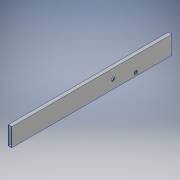
# Autodesk Inventor part: Side Extrusion
Saved by Autodesk Inventor 2019.4 (Build 234330000, 330)
## iProperties
Created: 2019-10-20
Part Number: Side Extrusion
Material: Aluminum 6061
Document SubType Name: Modeling
Designer: Mark
Density: 2.7 g/cm^3
Appearance: Aluminum - Flat
HoleDistanceX: 199.089 mm
Author: Mark
Autodesk Inventor part; units mm, degrees
ref_plane "YZ Plane" through (0, 0, 0) normal (1, 0, 0) x (0, 1, 0)
ref_plane "XZ Plane" through (0, 0, 0) normal (0, 1, 0) x (-1, 0, 0)
ref_plane "XY Plane" through (0, 0, 0) normal (0, 0, 1) x (1, 0, 0)
sketch "Sketch1" plane through (0, 0, 0) normal (0, 0, 1) x (1, 0, 0)
  line L0 (-10, -50) -> (10, -50)
  line L1 (10, -50) -> (10, 50)
  line L2 (10, 50) -> (-10, 50)
  line L3 (-10, 50) -> (-10, -50)
  line L4 (-10, -50) -> (10, 50) construction
  line L5 (10, -50) -> (-10, 50) construction
  line L6 (-8, -48) -> (8, -48)
  line L7 (8, -48) -> (8, 48)
  line L8 (8, 48) -> (-8, 48)
  line L9 (-8, 48) -> (-8, -48)
  line L10 (-8, -48) -> (8, 48) construction
  line L11 (8, -48) -> (-8, 48) construction
  point P0 (0, 0)
  dimension "d0" = 20
  dimension "d1" = 100
  dimension "d2" = 16
  dimension "d3" = 96
  constraints: 24 end point, 4 midpoint, 4 parallel, 2 horizontal, 2 perpendicular
  measures "d0" distance of L2.end L1.end
  measures "d1" distance of L1.end L0.end
  measures "d2" distance of L8.end L7.end
  measures "d3" distance of L7.end L6.end
extrude "Extrusion1" add sketch "Sketch1" along normal blind 880
sketch "Sketch2" plane through (-10, -50, 0) normal (-1, 0, 0) x (0, 0, 1)
  circle A0 centre (199.089, 18.548) radius 9.8
  line L0 (0, 100) -> (880, 100) projected
  line L1 (0, 100) -> (0, 0) projected
  line L2 (0, 0) -> (880, 0) projected
  point P0 (0, 50)
  dimension "d6" = 19.6
  dimension "HoleDistanceX" = 199.089
  dimension "d11" = 18.548
  constraints: 1 centre point
  measures "d6" diameter of A0
  measures "HoleDistanceX" distance from line of L1 A0.centre
  measures "d11" distance from line of L2 A0.centre
extrude "Extrusion2" cut sketch "Sketch2" against normal blind 880
sketch "Sketch4" plane through (-10, -50, 0) normal (-1, 0, 0) x (0, 0, 1)
  circle A0 centre (113.659, 8.082) radius 4.5 construction
  circle A1 centre (199.089, 18.548) radius 8.3 construction
  line L0 (199.089, 18.548) -> (113.659, 8.082) construction
  line L1 (199.089, 18.548) -> (113.0203, 18.5713) construction
  circle A2 centre (113.0203, 18.5713) radius 4.5 construction
  arc A3 (113.0203, 18.5713) -> (113.659, 8.082) centre (199.089, 18.548) ccw construction
  arc A4 (113.0203, 18.5713) -> (113.659, 8.082) centre (199.089, 18.548) ccw construction
  arc A5 (108.5203, 18.5725) -> (109.1924, 7.5348) centre (199.089, 18.548) ccw
  arc A6 (117.5203, 18.5701) -> (118.1256, 8.6292) centre (199.089, 18.548) ccw
  arc A7 (117.5203, 18.5701) -> (108.5203, 18.5725) centre (113.0203, 18.5713) ccw
  arc A8 (109.1924, 7.5348) -> (118.1256, 8.6292) centre (113.659, 8.082) ccw
  line L2 (0, 0) -> (880, 0) projected
  line L3 (0, 100) -> (0, 0) projected
  point P0 (0, 50)
  dimension "d12" = 9
  dimension "d13" = 9
  dimension "d14" = 9
  dimension "d15" = 7
  dimension "d16" = 8.082
  dimension "d17" = 113.659
  constraints: 12 point on circle, 8 centre point, 4 end point, 4 tangent, 3 coincident, 1 equal length
  measures "d12" diameter of A0
  measures "d13" diameter of A2
  measures "d14" diameter of A7
  measures "d15" angle of L1 L0
  measures "d16" distance from line of L2 L0.end
  measures "d17" distance from line of L3 L0.end
extrude "Extrusion3" cut sketch "Sketch4" against normal blind 3
sketch "Sketch5" plane through (-10, -50, 0) normal (-1, 0, 0) x (0, 0, 1)
  circle A0 centre (324.061, 48.813) radius 30
  line L0 (0, 100) -> (0, 0) projected
  line L1 (0, 0) -> (880, 0) projected
  point P0 (0, 50)
  dimension "d20" = 60
  dimension "d21" = 324.061
  dimension "d22" = 48.813
  constraints: 1 centre point
  measures "d20" diameter of A0
  measures "d21" distance from line of L0 A0.centre
  measures "d22" distance from line of L1 A0.centre
extrude "Extrusion4" cut sketch "Sketch5" against normal blind 3
sketch "Sketch6" plane through (-10, -50, 0) normal (-1, 0, 0) x (0, 0, 1)
  line L0 (450, 75) -> (580, 75)
  line L1 (580, 75) -> (580, 25)
  line L2 (580, 25) -> (450, 25)
  line L3 (450, 25) -> (450, 75)
  line L4 (0, 100) -> (880, 100) projected
  line L5 (0, 100) -> (0, 0) projected
  point P0 (0, 50)
  dimension "d25" = 50
  dimension "d26" = 25
  dimension "d27" = 580
  dimension "d28" = 450
  constraints: 8 end point, 2 parallel, 1 horizontal, 1 perpendicular
  measures "d25" distance of L0.end L1.end
  measures "d26" distance between parallel lines of L4 L0
  measures "d27" distance between parallel lines of L5 L1
  measures "d28" distance between parallel lines of L5 L3
extrude "Extrusion5" cut sketch "Sketch6" against normal blind 3
sketch "Sketch7" plane through (8, -48, 0) normal (-1, 0, 0) x (0, 0, 1)
  circle A0 centre (324.061, 46.813) radius 30 projected
  circle A1 centre (324.061, 46.813) radius 9.8
  point P0 (0, 48)
  dimension "d31" = 19.6
  constraints: 1 centre point, 1 coincident
  measures "d31" diameter of A1
extrude "Extrusion6" cut sketch "Sketch7" against normal through all contours A1
body "Solid1"
